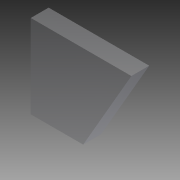
# Autodesk Inventor part: Top Plat
Saved by Autodesk Inventor 2015 (Build 190159000, 159)
## iProperties
Created: 2016-10-14
Part Number: Top Plat
Material: Polycarbonate, Clear
Document SubType Name: Modeling
Designer: James Yelland
Density: 1.2 g/cm^3
Appearance: Polycarbonate - Clear
Author: James Yelland
Autodesk Inventor part; units mm, degrees
ref_plane "YZ Plane" through (0, 0, 0) normal (1, 0, 0) x (0, 1, 0)
ref_plane "XZ Plane" through (0, 0, 0) normal (0, 1, 0) x (-1, 0, 0)
ref_plane "XY Plane" through (0, 0, 0) normal (0, 0, 1) x (1, 0, 0)
sketch "Sketch1" plane through (0, 0, 0) normal (0, 1, 0) x (-1, 0, 0)
  circle A0 centre (30.6147, -73.9104) radius 1.6
  circle A1 centre (-30.6147, -73.9104) radius 1.6
  circle A2 centre (30.6147, -73.9104) radius 1.6
  circle A3 centre (-30.6147, -73.9104) radius 1.6
  line L0 (103.5566, -2.5) -> (54.8095, -86.9325)
  line L1 (-54.8095, -86.9325) -> (-103.5566, -2.5)
  line L2 (-103.5566, 2.5) -> (-53.9434, 88.4327)
  line L3 (-49.6132, 90.9327) -> (49.6132, 90.9327)
  line L4 (53.9434, 88.4327) -> (103.5566, 2.5)
  arc A4 (48.3297, -88.9468) -> (54.8095, -86.9325) centre (50.4794, -84.4325) ccw
  arc A5 (-54.8095, -86.9325) -> (-48.3297, -88.9468) centre (-50.4794, -84.4325) ccw
  arc A6 (-103.5566, 2.5) -> (-103.5566, -2.5) centre (-99.2265, 0) ccw
  arc A7 (-49.6132, 90.9327) -> (-53.9434, 88.4327) centre (-49.6132, 85.9327) ccw
  arc A8 (53.9434, 88.4327) -> (49.6132, 90.9327) centre (49.6132, 85.9327) ccw
  arc A9 (103.5566, -2.5) -> (103.5566, 2.5) centre (99.2265, 0) ccw
  arc A10 (-43.8396, 80.9325) -> (-48.1698, 78.4325) centre (-43.8396, 75.9325) ccw
  arc A11 (-92.0094, 2.5) -> (-92.0094, -2.5) centre (-87.6793, 0) ccw
  line L5 (32.3518, -70.2624) -> (44.2883, -75.9464)
  arc A12 (44.2883, -75.9464) -> (50.7681, -73.9321) centre (46.4379, -71.4321) ccw
  line L6 (32.3518, -70.2624) -> (29.6432, -68.9726)
  line L7 (26.9776, -69.9184) -> (24.398, -75.3356)
  arc A13 (29.6432, -68.9726) -> (26.9776, -69.9184) centre (28.7834, -70.7783) ccw
  arc A14 (24.398, -75.3356) -> (25.3439, -78.0012) centre (26.2038, -76.1955) ccw
  circle A15 centre (-30.6147, -73.9104) radius 1.6
  circle A16 centre (-30.6147, -73.9104) radius 1.6
  line L8 (-32.3518, -70.2624) -> (-44.2883, -75.9464)
  arc A17 (-50.7681, -73.9321) -> (-44.2883, -75.9464) centre (-46.4379, -71.4321) ccw
  line L9 (-32.3518, -70.2624) -> (-29.6432, -68.9726)
  line L10 (-26.9776, -69.9184) -> (-24.398, -75.3356)
  arc A18 (-26.9776, -69.9184) -> (-29.6432, -68.9726) centre (-28.7834, -70.7783) ccw
  arc A19 (-25.3439, -78.0012) -> (-24.398, -75.3356) centre (-26.2038, -76.1955) ccw
  line L11 (48.3297, -88.9468) -> (25.3439, -78.0012)
  line L12 (-25.3439, -78.0012) -> (-48.3297, -88.9468)
  arc A20 (48.1698, 78.4325) -> (43.8396, 80.9325) centre (43.8396, 75.9325) ccw
  circle A21 centre (35.5991, 85.9437) radius 1.6
  circle A22 centre (-35.5945, 85.9327) radius 1.6
  circle A23 centre (92.2171, 12.1406) radius 1.6
  circle A24 centre (-92.2171, 12.1406) radius 1.6
  line L13 (-18.2679, -8.3495) -> (18.2679, -8.3495)
  line L14 (-92.0094, -2.5) -> (-50.7681, -73.9321)
  line L15 (50.7681, -73.9321) -> (70.8152, -39.2095)
  line L16 (59.1367, 11.2915) -> (33.0718, 11.2915)
  line L17 (59.1367, 11.2915) -> (68.2171, 11.2915)
  line L18 (-62.25, 35.5415) -> (-62.25, 17.0415)
  line L19 (-62.25, 17.0415) -> (-74.75, 17.0415)
  line L20 (-74.75, 17.0415) -> (-74.75, 35.5415)
  line L21 (-74.75, 35.5415) -> (-62.25, 35.5415)
  line L22 (-62.25, 35.5415) -> (-74.75, 17.0415) construction
  line L23 (-62.25, 17.0415) -> (-74.75, 35.5415) construction
  line L24 (30.4737, 9.7915) -> (20.866, -6.8495)
  line L25 (-92.0094, 2.5) -> (-87.7997, 9.7915)
  line L26 (-30.4737, 9.7915) -> (-20.866, -6.8495)
  arc A25 (33.0718, 11.2915) -> (30.4737, 9.7915) centre (33.0718, 8.2915) ccw
  arc A26 (64.417, 41.2915) -> (67.0151, 45.7915) centre (64.417, 44.2915) ccw
  arc A27 (30.4737, 42.7915) -> (33.0718, 41.2915) centre (33.0718, 44.2915) ccw
  arc A28 (18.2679, -8.3495) -> (20.866, -6.8495) centre (18.2679, -5.3495) ccw
  arc A29 (-20.866, -6.8495) -> (-18.2679, -8.3495) centre (-18.2679, -5.3495) ccw
  arc A30 (-30.4737, 9.7915) -> (-33.0718, 11.2915) centre (-33.0718, 8.2915) ccw
  arc A31 (-33.0718, 41.2915) -> (-30.4737, 42.7915) centre (-33.0718, 44.2915) ccw
  arc A32 (-18.2679, 60.9325) -> (-20.866, 59.4325) centre (-18.2679, 57.9325) ccw
  arc A33 (20.866, 59.4325) -> (18.2679, 60.9325) centre (18.2679, 57.9325) ccw
  arc A34 (-67.0151, 45.7915) -> (-64.417, 41.2915) centre (-64.417, 44.2915) ccw
  arc A35 (-85.2016, 11.2915) -> (-87.7997, 9.7915) centre (-85.2016, 8.2915) ccw
  line L27 (43.8396, 80.9325) -> (-43.8396, 80.9325)
  line L28 (-48.1698, 78.4325) -> (-67.0151, 45.7915)
  line L29 (-64.417, 41.2915) -> (-33.0718, 41.2915)
  line L30 (-30.4737, 42.7915) -> (-20.866, 59.4325)
  line L31 (-18.2679, 60.9325) -> (18.2679, 60.9325)
  line L32 (20.866, 59.4325) -> (30.4737, 42.7915)
  line L33 (33.0718, 41.2915) -> (64.417, 41.2915)
  line L34 (67.0151, 45.7915) -> (48.1698, 78.4325)
  line L35 (-56.75, 35.5415) -> (-56.75, 17.0415)
  line L36 (-56.75, 17.0415) -> (-44.25, 17.0415)
  line L37 (-44.25, 17.0415) -> (-44.25, 35.5415)
  line L38 (-44.25, 35.5415) -> (-56.75, 35.5415)
  line L39 (-56.75, 35.5415) -> (-44.25, 17.0415) construction
  line L40 (-56.75, 17.0415) -> (-44.25, 35.5415) construction
  circle A36 centre (-55.4009, 75.9081) radius 1.6
  circle A37 centre (55.3868, 75.9325) radius 1.6
  line L41 (-17.5, 81.9327) -> (17.5, 81.9327)
  line L42 (17.5, 81.9327) -> (17.5, 89.9327)
  line L43 (17.5, 89.9327) -> (-17.5, 89.9327)
  line L44 (-17.5, 89.9327) -> (-17.5, 81.9327)
  circle A38 centre (-12, 85.9327) radius 1.45
  circle A39 centre (12, 85.9327) radius 1.45
  line L45 (0, 90.9327) -> (0, 89.9327)
  line L46 (0, 89.9327) -> (0, 81.9327)
  line L47 (-74.2171, -27.8594) -> (-74.2171, 7.1406)
  line L48 (-74.2171, 7.1406) -> (-82.2171, 7.1406)
  line L49 (-82.2171, 7.1406) -> (-82.2171, -27.8594)
  line L50 (-82.2171, -27.8594) -> (-74.2171, -27.8594)
  circle A40 centre (-78.2171, -22.3594) radius 1.45
  circle A41 centre (-78.2171, 1.6406) radius 1.45
  line L51 (-82.2171, -10.3594) -> (-74.2171, -10.3594)
  line L52 (82.2171, -27.8594) -> (82.2171, 7.1406)
  line L53 (82.2171, 7.1406) -> (74.2171, 7.1406)
  line L54 (74.2171, 7.1406) -> (74.2171, -27.8594)
  line L55 (74.2171, -27.8594) -> (82.2171, -27.8594)
  circle A42 centre (78.2171, -22.3594) radius 1.45
  circle A43 centre (78.2171, 1.6406) radius 1.45
  line L56 (74.2171, -10.3594) -> (82.2171, -10.3594)
  line L57 (-71.6147, -49.9104) -> (-36.6147, -49.9104)
  line L58 (-36.6147, -49.9104) -> (-36.6147, -41.9104)
  line L59 (-36.6147, -41.9104) -> (-71.6147, -41.9104)
  line L60 (-71.6147, -41.9104) -> (-71.6147, -49.9104)
  circle A44 centre (-66.1147, -45.9104) radius 1.45
  circle A45 centre (-42.1147, -45.9104) radius 1.45
  line L61 (-54.1147, -41.9104) -> (-54.1147, -49.9104)
  line L62 (-30.6147, -73.9104) -> (-35.6147, -73.9104)
  line L63 (-35.6147, -73.9104) -> (-35.6147, -45.9104)
  line L64 (-36.6147, -45.9104) -> (-35.6147, -45.9104)
  line L65 (92.2171, 12.1406) -> (97.2171, 12.1406) construction
  line L66 (-92.2171, 12.1406) -> (-92.2171, 7.1406)
  line L67 (-92.2171, 12.1406) -> (-87.2171, 12.1406) construction
  line L68 (-92.2171, 7.1406) -> (-82.2171, 7.1406)
  line L69 (74.2171, -10.3594) -> (71.2171, -10.3594)
  line L70 (71.2171, -10.3594) -> (71.2171, 8.2915)
  line L71 (71.2171, -10.3594) -> (71.2171, -37.7095)
  line L72 (-74.2171, -10.3594) -> (-71.2171, -10.3594)
  line L73 (-71.2171, -10.3594) -> (-71.2171, 11.2915)
  line L74 (-71.2171, -10.3594) -> (-49.5662, -10.3594) construction
  line L75 (-71.2171, -10.3594) -> (-71.2171, -38.5133)
  line L76 (-71.2171, -10.3594) -> (-43.0632, -10.3594) construction
  arc A46 (70.8152, -39.2095) -> (71.2171, -37.7095) centre (68.2171, -37.7095) ccw
  arc A47 (71.2171, 8.2915) -> (68.2171, 11.2915) centre (68.2171, 8.2915) ccw
  line L77 (-54.1147, -41.9104) -> (-54.1147, -38.9104)
  line L78 (-54.1147, -38.9104) -> (-70.9879, -38.9104)
  line L79 (-54.1147, -49.9104) -> (-54.1147, -52.9104)
  line L80 (-54.1147, -52.9104) -> (-62.905, -52.9104)
  line L81 (-36.6147, -45.9104) -> (-33.6147, -45.9104)
  line L82 (-33.6147, -45.9104) -> (-33.6147, -52.9104)
  point P0 (105, 0)
  point P1 (52.5, -90.9327)
  point P2 (-105, 0)
  point P3 (-52.5, 90.9327)
  point P4 (52.5, 90.9327)
  point P5 (-93.4528, 0)
  point P6 (-46.7264, 80.9325)
  point P7 (46.7264, 80.9325)
  point P8 (-5, -80.9325)
  point P9 (5, -80.9325)
  point P10 (92.0094, -2.5)
  point P11 (69.6132, 41.2915)
  point P12 (86.9337, 11.2915)
  point P13 (-69.6132, 41.2915)
  point P14 (-86.9337, 11.2915)
  point P15 (85.2016, 11.2915)
  point P16 (0, 60.9325)
  point P17 (0, -8.3495)
  point P18 (71.2171, -38.5133)
  dimension "d148" = 5
  dimension "d150" = 2
  dimension "d234" = 18.5
  dimension "d249" = 35
  dimension "d250" = 8
  dimension "d252" = 2.9
  dimension "d254" = 2.9
  dimension "d255" = 1
  dimension "d256" = 35
  dimension "d257" = 8
  dimension "d258" = 2.9
  dimension "d259" = 2.9
  dimension "d261" = 35
  dimension "d262" = 8
  dimension "d263" = 2.9
  dimension "d264" = 2.9
  dimension "d266" = 35
  dimension "d267" = 8
  dimension "d268" = 2.9
  dimension "d269" = 2.9
  dimension "d271" = 5
  dimension "d272" = 28
  dimension "d273" = 1
  dimension "d277" = 5
  dimension "d278" = 90
  dimension "d279" = 10
  dimension "d280" = 3
  dimension "d281" = 3
  dimension "d282" = 90
  dimension "d283" = 90
  dimension "d284" = 3
  dimension "d285" = 3
  dimension "d286" = 3
  dimension "d287" = 3
  dimension "d288" = 90
  constraints: 166 end point, 57 point on circle, 48 centre point, 21 point on line, 16 parallel, 13 perpendicular, 12 midpoint, 12 tangent, 9 horizontal, 4 vertical, 3 coincident, 1 equal radius
  measures "d148" radius of A12
  measures "d150" radius of A13
  measures "d234" distance of L18.start L18.end
  measures "d249" distance of L41.start L41.end
  measures "d250" distance of L42.end L41.end
  measures "d252" diameter of A38
  measures "d254" diameter of A39
  measures "d255" distance of L45.start L45.end
  measures "d256" distance of L47.start L48.start
  measures "d257" distance of L48.end L48.start
  measures "d258" diameter of A40
  measures "d259" diameter of A41
  measures "d261" distance of L52.start L53.start
  measures "d262" distance of L53.end L53.start
  measures "d263" diameter of A42
  measures "d264" diameter of A43
  measures "d266" distance of L57.start L58.start
  measures "d267" distance of L58.end L58.start
  measures "d268" diameter of A44
  measures "d269" diameter of A45
  measures "d271" distance of L62.start L62.end
  measures "d272" distance of L62.end L63.end
  measures "d273" distance of L64.start L64.end
  measures "d277" distance of L66.start L66.end
  measures "d278" angle of L66 L67
  measures "d279" distance of L66.end L68.end
  measures "d280" distance of L56.start L69.end
  measures "d281" distance of L51.end L72.end
  measures "d282" angle of L74 L73
  measures "d283" angle of L75 L76
  measures "d284" radius of A46
  measures "d285" distance of L61.start L77.end
  measures "d286" distance of L61.end L79.end
  measures "d287" distance of L64.start L81.end
  measures "d288" angle of L81 L82
extrude "Extrusion2" add sketch "Sketch1" along normal blind 3 contours L14 L57 L79 L80 | L14 A44 L59 L61 L57 | L59 L14 L78 L77 | L14 A44 picked at (-66.6874, -45.6933)
body "Solid2"
